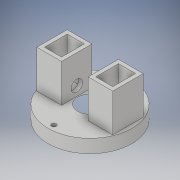
# Autodesk Inventor part: funil
Saved by Autodesk Inventor 2017 (Build 210142000, 142)
## iProperties
Created: 2017-03-09
Part Number: funil
Material: Generic
Document SubType Name: Modeling
Designer: vitor
Density: 1 g/cm^3
Appearance: Default
Author: vitor
Autodesk Inventor part; units mm, degrees
ref_plane "YZ Plane" through (0, 0, 0) normal (1, 0, 0) x (0, 1, 0)
ref_plane "XZ Plane" through (0, 0, 0) normal (0, 1, 0) x (-1, 0, 0)
ref_plane "XY Plane" through (0, 0, 0) normal (0, 0, 1) x (1, 0, 0)
sketch "Sketch1" plane through (0, 0, 0) normal (0, 1, 0) x (-1, 0, 0)
  circle A0 centre (0, 0) radius 22
  dimension "d0" = 44
  constraints: 1 centre point, 1 coincident
  measures "d0" diameter of A0
extrude "Extrusion1" add sketch "Sketch1" along normal blind 7
sketch "Sketch3" plane through (0, 0, 0) normal (0, -1, 0) x (1, 0, 0)
  circle A0 centre (0, 0) radius 15
  dimension "d4" = 30
  constraints: 1 centre point, 1 coincident
  measures "d4" diameter of A0
extrude "Extrusion2" [suppressed]
sketch "Sketch4" plane through (0, 2, 0) normal (0, -1, 0) x (1, 0, 0)
  circle A0 centre (0, 0) radius 12
  dimension "d11" = 24
  constraints: 1 centre point, 1 coincident
  measures "d11" diameter of A0
extrude "Extrusion3" [suppressed]
sketch "Sketch5" plane through (0, 4, 0) normal (0, -1, 0) x (1, 0, 0)
  circle A0 centre (0, 0) radius 10
  dimension "d14" = 20
  constraints: 1 centre point, 1 coincident
  measures "d14" diameter of A0
extrude "Extrusion4" [suppressed]
sketch "Sketch6" plane through (0, 6, 0) normal (0, -1, 0) x (1, 0, 0)
  circle A0 centre (0, 0) radius 8.5
  dimension "d17" = 17
  constraints: 1 centre point, 1 coincident
  measures "d17" diameter of A0
extrude "Extrusion5" [suppressed]
sketch "Sketch7" plane through (0, 8, 0) normal (0, -1, 0) x (1, 0, 0)
  circle A0 centre (0, 0) radius 7
  dimension "d20" = 14
  constraints: 1 centre point, 1 coincident
  measures "d20" diameter of A0
extrude "Extrusion6" [suppressed]
sketch "Sketch9" plane through (0, 7, 0) normal (0, 1, 0) x (1, 0, 0)
  line L0 (20, 8) -> (7, 8)
  line L1 (7, 8) -> (7, -8)
  line L2 (7, -8) -> (20, -8)
  line L3 (20, -8) -> (20, 8)
  line L4 (-20, 8) -> (-7, 8)
  line L5 (-7, 8) -> (-7, -8)
  line L6 (-7, -8) -> (-20, -8)
  line L7 (-20, -8) -> (-20, 8)
  line L8 (18, 6) -> (9, 6)
  line L9 (9, 6) -> (9, -6)
  line L10 (9, -6) -> (18, -6)
  line L11 (18, -6) -> (18, 6)
  line L12 (-9, 6) -> (-18, 6)
  line L13 (-18, 6) -> (-18, -6)
  line L14 (-18, -6) -> (-9, -6)
  line L15 (-9, -6) -> (-9, 6)
  point P0 (0, 0)
  point P1 (7, 0)
  point P2 (-7, 0)
  point P3 (9, 0)
  point P4 (-9, 0)
  dimension "d29" = 13
  dimension "d30" = 16
  dimension "d31" = 7
  dimension "d32" = 13
  dimension "d33" = 16
  dimension "d34" = 7
  dimension "d35" = 9
  dimension "d36" = 12
  dimension "d37" = 2
  dimension "d38" = 9
  dimension "d39" = 12
  dimension "d40" = 2
  constraints: 32 end point, 8 parallel, 4 horizontal, 4 horizontal alignment, 4 midpoint, 4 perpendicular
  measures "d29" distance of L2.end L1.end
  measures "d30" distance of L1.end L0.end
  measures "d31" distance from line of point (0, 0) L1
  measures "d32" distance of L5.end L6.end
  measures "d33" distance of L4.end L5.end
  measures "d34" distance from line of point (0, 0) L5
  measures "d35" distance of L10.end L9.end
  measures "d36" distance of L9.end L8.end
  measures "d37" distance between parallel lines of L1 L9
  measures "d38" distance of L14.end L13.end
  measures "d39" distance of L13.end L12.end
  measures "d40" distance between parallel lines of L5 L15
extrude "Extrusion8" add sketch "Sketch9" along normal blind 20
sketch "Sketch8" plane through (0, 0, 0) normal (0, -1, 0) x (1, 0, 0)
  circle A0 centre (0, 19) radius 1.25
  circle A1 centre (0, -19) radius 1.25
  point P0 (0, 0)
  dimension "d23" = 2.5
  dimension "d24" = 2.5
  dimension "d25" = 19
  dimension "d26" = 19
  constraints: 2 centre point
  measures "d23" diameter of A0
  measures "d24" diameter of A1
  measures "d25" distance of A0.centre point (0, 0)
  measures "d26" distance of A1.centre point (0, 0)
extrude "Extrusion7" cut sketch "Sketch8" against normal blind 14
sketch "Sketch10" plane through (-7, 10, 0) normal (1, 0, 0) x (0, 0, -1)
  circle A0 centre (0, 2) radius 3
  line L0 (-8, 17) -> (8, 17) projected
  point P0 (0, -10)
  dimension "d43" = 6
  dimension "d44" = 15
  constraints: 1 centre point
  measures "d43" diameter of A0
  measures "d44" distance from line of L0 A0.centre
extrude "Extrusion9" cut sketch "Sketch10" against normal blind 2
sketch "Sketch11" plane through (7, 7, -8) normal (-1, 0, 0) x (0, 0, 1)
  circle A0 centre (8, 5) radius 2
  line L0 (0, 20) -> (16, 20) projected
  point P0 (8, -7)
  dimension "d47" = 4
  dimension "d48" = 15
  constraints: 1 centre point
  measures "d47" diameter of A0
  measures "d48" distance from line of L0 A0.centre
extrude "Extrusion10" cut sketch "Sketch11" against normal blind 2
sketch "Sketch12" plane through (0, 0, 0) normal (1, 0, 0) x (0, 1, 0)
  line L0 (7, 6.5) -> (0, 17)
  line L1 (7, 0) -> (7, 6.5)
  line L2 (7, 0) -> (0, 0)
  line L3 (0, 0) -> (0, 17)
  line L4 (0, 22) -> (0, -22) projected
  dimension "d54" = 6.5
  dimension "d55" = 17
  dimension "d56" = 7
  constraints: 8 end point, 1 collinear, 1 horizontal
  measures "d54" distance of L1.start L0.start
  measures "d55" distance of L2.end L0.end
  measures "d56" distance of L1.start L2.end
revolve "Revolution1" cut sketch "Sketch12" angle 360 about axis through (0, 7, 0) along (0, -1, 0)
body "Solid1"
